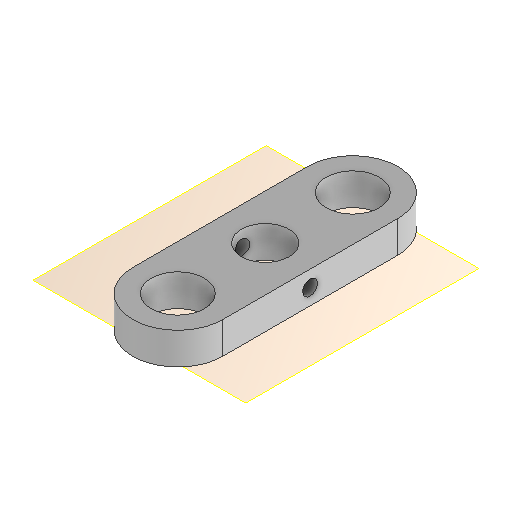
# Autodesk Inventor part: 40_XYZstage_micrometer_motorized_nema8_samplemount_lightsheet_syringemount_screwed
Saved by Autodesk Inventor 2024.1 (Build 281209000, 209)
## iProperties
Created: 2024-03-18
Part Number: 40_XYZstage_micrometer_motorized_nema8_samplemount_lightsheet_syringemount_screwed
Material: Generisch
Document SubType Name: Modeling
Designer: diederichbenedict
Density: 1 g/cm^3
Appearance: Vorgabe
Author: diederichbenedict
Autodesk Inventor part; units mm, degrees
ref_plane "YZ Plane" through (0, 0, 0) normal (1, 0, 0) x (0, 1, 0)
ref_plane "XZ Plane" through (0, 0, 0) normal (0, 1, 0) x (-1, 0, 0)
ref_plane "XY Plane" through (0, 0, 0) normal (0, 0, 1) x (1, 0, 0)
ref_plane "Arbeitsebene1" through (0, 0, 0) normal (0, 0, 1) x (1, 0, 0)
sketch "Skizze1" plane through (0, 0, 0) normal (0, 0, 1) x (1, 0, 0)
  circle A0 centre (-13, -20) radius 11 projected
  circle A1 centre (-13, -36.5) radius 2 projected
  circle A2 centre (-13, -3.5) radius 2 projected
  line L0 (0, 0) -> (0, -9.8388) projected
  line L1 (-29, 0) -> (0, 0) projected
  line L2 (-33, -4) -> (-29, 0) projected
  line L3 (-33, -4) -> (-33, -36) projected
  line L4 (-29, -40) -> (-33, -36) projected
  line L5 (0, -40) -> (-29, -40) projected
  line L6 (0, -30.1612) -> (0, -40) projected
  arc A3 (0, -30.1612) -> (0, -9.8388) centre (-13, -20) ccw projected
  circle A4 centre (-13, -3.5) radius 5
  circle A5 centre (-13, -36.5) radius 5
  circle A6 centre (-13, -20) radius 4.5
  line L7 (-13, -3.5) -> (-13, -36.5) construction
  line L8 (-21.5, -3.5) -> (-21.5, -36.5)
  line L9 (-4.5, -36.5) -> (-4.5, -3.5)
  arc A7 (-4.5, -3.5) -> (-21.5, -3.5) centre (-13, -3.5) ccw
  arc A8 (-21.5, -36.5) -> (-4.5, -36.5) centre (-13, -36.5) ccw
  point P0 (-13, -20)
  dimension "d0" = 10
  dimension "d1" = 10
  dimension "d2" = 9
  dimension "d3" = 17
  constraints: 8 end point, 5 centre point, 4 point on circle, 4 tangent, 3 coincident, 1 midpoint, 1 parallel, 1 vertical
  measures "d0" diameter of A4
  measures "d1" diameter of A5
  measures "d2" diameter of A6
  measures "d3" diameter of A8
extrude "Extrusion1" add sketch "Skizze1" along normal blind 6 contours L9 A0 L8 | A0 L8 A7 L1 A4 L9 | L9 A8 L5 A5 L8 A0 | L1 A4 A7 | A8 L5 A5
sketch "Skizze2" plane through (-21.5, -36.5, 0) normal (-1, 0, 0) x (0, 0, 1)
  line L0 (6, 21) -> (0, 21) projected
  line L1 (6, 12) -> (0, 12) projected
  circle A0 centre (3, 16.4602) radius 1.4
  point P0 (0, 36.5)
  dimension "d6" = 2.8
  constraints: 1 centre point
  measures "d6" diameter of A0
extrude "Extrusion2" cut sketch "Skizze2" against normal through all
